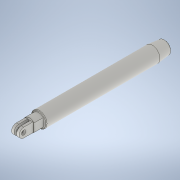
# Autodesk Inventor part: Kolbenstange
Saved by Autodesk Inventor 2020.3 (Build 243373000, 373)
## iProperties
Created: 2021-05-20
Part Number: Kolbenstange
Material: Stahl AISI 4130
Document SubType Name: Modeling
Designer: Preuß P. Ch.
Density: 7.85 g/cm^3
Appearance: Stahl
Author: Preuß P. Ch.
Autodesk Inventor part; units mm, degrees
ref_plane "YZ Plane" through (0, 0, 0) normal (1, 0, 0) x (0, 1, 0)
ref_plane "XZ Plane" through (0, 0, 0) normal (0, 1, 0) x (-1, 0, 0)
ref_plane "XY Plane" through (0, 0, 0) normal (0, 0, 1) x (1, 0, 0)
sketch "Skizze1" plane through (0, 0, 0) normal (0, 0, 1) x (1, 0, 0)
  line L0 (0, 0) -> (0, 20.7958)
  line L1 (0, 20.7958) -> (40, 25)
  line L2 (40, 25) -> (405, 25)
  line L3 (405, 25) -> (405, 0)
  line L4 (405, 0) -> (0, 0)
  line L5 (405, 0) -> (435, 0)
  line L6 (435, 0) -> (435, 20)
  line L7 (435, 20) -> (405, 20)
  line L8 (405, 20) -> (405, 0)
  line L9 (435, 15) -> (480, 15)
  line L10 (480, 15) -> (480, -15)
  line L11 (480, -15) -> (435, -15)
  line L12 (435, -15) -> (435, 15)
  dimension "d0" = 480
  dimension "d1" = 30
  dimension "d2" = 40
  dimension "d3" = 50
  dimension "d4" = 6
  dimension "d5" = 40
  dimension "d6" = 30
  dimension "d7" = 75
  constraints: 26 end point, 5 perpendicular, 4 parallel, 2 horizontal, 1 midpoint, 1 vertical
  measures "d0" distance between parallel lines of L10 L0
  measures "d1" distance of L9.end L10.end
  measures "d2" diameter of L7 L4
  measures "d3" diameter of L2 L4
  measures "d4" angle of L1 L2
  measures "d5" distance from line of L1.end L0
  measures "d6" distance of L6.end L7.end
  measures "d7" distance between parallel lines of L10 L3
revolve "Umdrehung1" add sketch "Skizze1" angle 360 about axis through (405, 0, 0) along (-1, 0, 0) contours L0 L1 L2 L3 L4 | L3 L7 L6 L5
extrude "Extrusion1" add sketch "Skizze1" along normal mid plane 24 contours L6 L9 L10 L11 L12
full round fillet "Rundung1" first side at (450, 15, 4) centre faces at (480, 5, 4) second side at (450, -15, -4)
extrude "Extrusion2" cut sketch "Skizze1" along normal mid plane 8 contours L6 L9 L10 L11 L12
sketch "Skizze2" plane through (0, 0, 12) normal (0, 0, 1) x (1, 0, 0)
  arc A0 (465, -15) -> (465, 15) centre (465, 0) ccw projected
  point P0 (0, 0)
  constraints: 1 coincident
hole "Bohrung1" at (465, 0, 12) direction (0, 0, -1) diameter 14 end through all
sketch "Skizze3" plane through (435, 0, 0) normal (1, 0, 0) x (0, 0, -1)
  line L0 (-15, -20) -> (-20, -20)
  line L1 (-20, -20) -> (-20, 20)
  line L2 (-20, 20) -> (-15, 20)
  line L3 (-15, 20) -> (-15, -20)
  line L4 (20, -20) -> (15, -20)
  line L5 (15, -20) -> (15, 20)
  line L6 (15, 20) -> (20, 20)
  line L7 (20, 20) -> (20, -20)
  circle A0 centre (0, 0) radius 20 projected
  point P0 (-15, -13.2288)
  point P1 (-20, 0)
  point P2 (-15, 13.2288)
  dimension "d20" = 30
  constraints: 16 end point, 6 tangent, 4 parallel, 2 horizontal, 2 perpendicular, 1 collinear
  measures "d20" distance between parallel lines of L3 L5
extrude "Extrusion3" cut sketch "Skizze3" against normal up to surface (30 mm away) contours L0 L1 A0 L3 | A0 L3 | L1 L2 L3 A0 | A0 L7 L4 L5 | L5 A0 | L5 L6 L7 A0
chamfer "Fase1" distance 2 angle 45 2 edges at (405, -25, 0) (0, -20.7958, 0)
